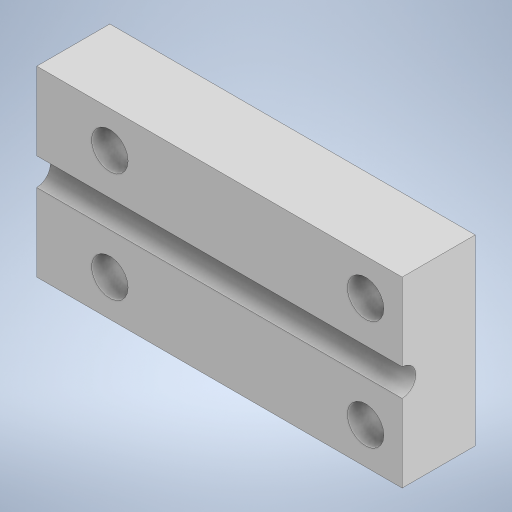
# Autodesk Inventor part: fiber_top
Saved by Autodesk Inventor 2024 (Build 280153000, 153)
## iProperties
Created: 2023-11-01
Part Number: fiber_top
Material: Generic
Document SubType Name: Modeling
Designer: toybox
Density: 1 g/cm^3
Appearance: Default
Author: toybox
Autodesk Inventor part; units mm, degrees
ref_plane "YZ Plane" through (0, 0, 0) normal (1, 0, 0) x (0, 1, 0)
ref_plane "XZ Plane" through (0, 0, 0) normal (0, 1, 0) x (-1, 0, 0)
ref_plane "XY Plane" through (0, 0, 0) normal (0, 0, 1) x (1, 0, 0)
sketch "Sketch3" plane through (0, 0, 0) normal (0, 0, 1) x (1, 0, 0)
  line L0 (-10, 5) -> (10, 5)
  line L1 (10, 5) -> (10, -5)
  line L2 (10, -5) -> (-10, -5)
  line L3 (-10, -5) -> (-10, 5)
  line L4 (-10, 5) -> (10, -5) construction
  line L5 (10, 5) -> (-10, -5) construction
  point P0 (0, 0)
  dimension "d5" = 20
  dimension "d6" = 10
  constraints: 12 end point, 2 midpoint, 2 parallel, 1 horizontal, 1 perpendicular
  measures "d5" distance of L1.end L2.end
  measures "d6" distance of L0.end L1.end
extrude "Extrusion2" add sketch "Sketch3" along normal blind 4
sketch "Sketch4" plane through (10, -5, 0) normal (1, 0, 0) x (0, 0, -1)
  circle A0 centre (-4, 5) radius 0.75
  point P0 (0, 5)
  dimension "d10" = 1.5
  constraints: 1 centre point
  measures "d10" diameter of A0
extrude "Extrusion3" cut sketch "Sketch4" against normal through all
sketch "Sketch5" plane through (0, 0, 4) normal (0, 0, 1) x (1, 0, 0)
  circle A0 centre (8, 3) radius 1
  circle A1 centre (8, -3) radius 1
  circle A2 centre (-6, 3) radius 1
  circle A3 centre (-6, -3) radius 1
  point P0 (0, 0)
  dimension "d17" = 2
  dimension "d16" = 2
  dimension "d15" = 2
  dimension "d14" = 2
  constraints: 4 centre point
  measures "d17" diameter of A0
  measures "d16" diameter of A1
  measures "d15" diameter of A2
  measures "d14" diameter of A3
extrude "Extrusion4" cut sketch "Sketch5" against normal through all
sketch "Sketch6" plane through (0, 0, 0) normal (0, 0, -1) x (-1, 0, 0)
  line L0 (-8.1739, 1.5824) -> (1.6987, 1.5824) construction
  line L1 (1.6987, 1.5824) -> (1.6987, -1.5298) construction
  line L2 (1.6987, -1.5298) -> (-8.1739, -1.5298) construction
  line L3 (-8.1739, -1.5298) -> (-8.1739, 1.5824) construction
  line L4 (-7.2861, -1.2743) -> (-7.2861, 1.3892)
  spline S0 degree 2 poles (-7.2861, 1.3892) (-7.2861, 1.5824) (-7.09, 1.5824) knots 0 0 0 1 1 1
  line L5 (-7.09, 1.5824) -> (-5.9053, 1.5824)
  spline S1 degree 2 poles (-5.9053, 1.5824) (-5.7093, 1.5824) (-5.7093, 1.3892) knots 0 0 0 1 1 1
  spline S2 degree 2 poles (-5.7093, 1.3892) (-5.7093, 1.1931) (-5.9053, 1.1931) knots 0 0 0 1 1 1
  line L6 (-5.9053, 1.1931) -> (-6.894, 1.1931)
  line L7 (-6.894, 1.1931) -> (-6.894, 0.3977)
  line L8 (-6.894, 0.3977) -> (-5.9053, 0.3977)
  spline S3 degree 2 poles (-5.9053, 0.3977) (-5.7093, 0.3977) (-5.7093, 0.2045) knots 0 0 0 1 1 1
  spline S4 degree 2 poles (-5.7093, 0.2045) (-5.7093, 0.0084) (-5.9053, 0.0084) knots 0 0 0 1 1 1
  line L9 (-5.9053, 0.0084) -> (-6.894, 0.0084)
  line L10 (-6.894, 0.0084) -> (-6.894, -1.2743)
  spline S5 degree 2 poles (-6.894, -1.2743) (-6.894, -1.4704) (-7.09, -1.4704) knots 0 0 0 1 1 1
  spline S6 degree 2 poles (-7.09, -1.4704) (-7.2861, -1.4704) (-7.2861, -1.2743) knots 0 0 0 1 1 1
  spline S7 degree 2 poles (-3.3734, 0.5014) (-3.3734, 0.6918) (-3.1774, 0.6918) knots 0 0 0 1 1 1
  spline S8 degree 2 poles (-3.1774, 0.6918) (-2.9813, 0.6918) (-2.9813, 0.5014) knots 0 0 0 1 1 1
  line L11 (-2.9813, 0.5014) -> (-2.9813, -1.2743)
  spline S9 degree 2 poles (-2.9813, -1.2743) (-2.9813, -1.4704) (-3.1774, -1.4704) knots 0 0 0 1 1 1
  spline S10 degree 2 poles (-3.1774, -1.4704) (-3.3734, -1.4704) (-3.3734, -1.2743) knots 0 0 0 1 1 1
  line L12 (-3.3734, -1.2743) -> (-3.3734, 0.5014)
  line L13 (-3.3734, 1.2379) -> (-3.3734, 1.3864)
  spline S11 degree 2 poles (-3.3734, 1.3864) (-3.3734, 1.5796) (-3.1774, 1.5796) knots 0 0 0 1 1 1
  spline S12 degree 2 poles (-3.1774, 1.5796) (-2.9813, 1.5796) (-2.9813, 1.3864) knots 0 0 0 1 1 1
  line L14 (-2.9813, 1.3864) -> (-2.9813, 1.2379)
  spline S13 degree 2 poles (-2.9813, 1.2379) (-2.9813, 1.0447) (-3.1774, 1.0447) knots 0 0 0 1 1 1
  spline S14 degree 2 poles (-3.1774, 1.0447) (-3.3734, 1.0447) (-3.3734, 1.2379) knots 0 0 0 1 1 1
  line L15 (0.9313, 0.0588) -> (0.9313, -0.8318)
  spline S15 degree 2 poles (0.9313, -0.8318) (0.9313, -1.1007) (0.5616, -1.4704) (0.2927, -1.4704) knots 0 0 0 1 2 2 2
  line L16 (0.2927, -1.4704) -> (-0.4467, -1.4704)
  spline S16 degree 2 poles (-0.4467, -1.4704) (-0.6427, -1.4704) (-0.6427, -1.2743) knots 0 0 0 1 1 1
  line L17 (-0.6427, -1.2743) -> (-0.6427, 1.3864)
  spline S17 degree 2 poles (-0.6427, 1.3864) (-0.6427, 1.5796) (-0.4467, 1.5796) knots 0 0 0 1 1 1
  spline S18 degree 2 poles (-0.4467, 1.5796) (-0.2506, 1.5796) (-0.2506, 1.3864) knots 0 0 0 1 1 1
  line L18 (-0.2506, 1.3864) -> (-0.2506, 0.6946)
  line L19 (-0.2506, 0.6946) -> (0.2927, 0.6946)
  spline S19 degree 2 poles (0.2927, 0.6946) (0.6652, 0.6946) (0.8473, 0.3781) knots 0 0 0 1 1 1
  spline S20 degree 2 poles (0.8473, 0.3781) (0.9313, 0.2297) (0.9313, 0.0588) knots 0 0 0 1 1 1
  line L20 (0.2927, 0.3053) -> (-0.2506, 0.3053)
  line L21 (-0.2506, 0.3053) -> (-0.2506, -1.0811)
  line L22 (-0.2506, -1.0811) -> (0.2927, -1.0811)
  spline S21 degree 2 poles (0.2927, -1.0811) (0.3935, -1.0811) (0.5392, -0.9354) (0.5392, -0.829) knots 0 0 0 1 2 2 2
  line L23 (0.5392, -0.829) -> (0.5392, 0.056)
  spline S22 degree 2 poles (0.5392, 0.056) (0.5392, 0.1625) (0.3963, 0.3053) (0.2927, 0.3053) knots 0 0 0 1 2 2 2
  line L24 (3.071, -0.5825) -> (3.071, -0.829)
  spline S23 degree 2 poles (3.071, -0.829) (3.071, -0.9326) (3.2195, -1.0811) (3.3203, -1.0811) knots 0 0 0 1 2 2 2
  line L25 (3.3203, -1.0811) -> (4.0597, -1.0811)
  spline S24 degree 2 poles (4.0597, -1.0811) (4.2558, -1.0811) (4.2558, -1.2743) knots 0 0 0 1 1 1
  spline S25 degree 2 poles (4.2558, -1.2743) (4.2558, -1.4704) (4.0597, -1.4704) knots 0 0 0 1 1 1
  line L26 (4.0597, -1.4704) -> (3.3203, -1.4704)
  spline S26 degree 2 poles (3.3203, -1.4704) (3.0486, -1.4704) (2.6789, -1.1007) (2.6789, -0.8318) knots 0 0 0 1 2 2 2
  line L27 (2.6789, -0.8318) -> (2.6789, -0.0924)
  spline S27 degree 2 poles (2.6789, -0.0924) (2.6789, 0.2325) (3.1383, 0.6918) (3.4659, 0.6918) knots 0 0 0 1 2 2 2
  spline S28 degree 2 poles (3.4659, 0.6918) (3.7992, 0.6918) (4.2558, 0.2381) (4.2558, -0.0924) knots 0 0 0 1 2 2 2
  line L28 (4.2558, -0.0924) -> (4.2558, -0.5825)
  line L29 (4.2558, -0.5825) -> (3.071, -0.5825)
  spline S29 degree 2 poles (3.4659, 0.3053) (3.3035, 0.3053) (3.071, 0.0728) (3.071, -0.0896) knots 0 0 0 1 2 2 2
  line L30 (3.071, -0.0896) -> (3.071, -0.1932)
  line L31 (3.071, -0.1932) -> (3.8636, -0.1932)
  line L32 (3.8636, -0.1932) -> (3.8636, -0.0896)
  spline S30 degree 2 poles (3.8636, -0.0896) (3.8636, 0.0728) (3.6312, 0.3053) (3.4659, 0.3053) knots 0 0 0 1 2 2 2
  spline S31 degree 2 poles (6.149, 0.5014) (6.149, 0.6946) (6.3451, 0.6946) knots 0 0 0 1 1 1
  line L33 (6.3451, 0.6946) -> (7.2329, 0.6946)
  spline S32 degree 2 poles (7.2329, 0.6946) (7.429, 0.6946) (7.429, 0.5014) knots 0 0 0 1 1 1
  line L34 (7.429, 0.5014) -> (7.429, 0.2045)
  spline S33 degree 2 poles (7.429, 0.2045) (7.429, 0.0084) (7.2329, 0.0084) knots 0 0 0 1 1 1
  spline S34 degree 2 poles (7.2329, 0.0084) (7.0369, 0.0084) (7.0369, 0.2045) knots 0 0 0 1 1 1
  line L35 (7.0369, 0.2045) -> (7.0369, 0.3053)
  line L36 (7.0369, 0.3053) -> (6.5412, 0.3053)
  line L37 (6.5412, 0.3053) -> (6.5412, -1.2743)
  spline S35 degree 2 poles (6.5412, -1.2743) (6.5412, -1.4704) (6.3451, -1.4704) knots 0 0 0 1 1 1
  spline S36 degree 2 poles (6.3451, -1.4704) (6.149, -1.4704) (6.149, -1.2743) knots 0 0 0 1 1 1
  line L38 (6.149, -1.2743) -> (6.149, 0.5014)
  point P0 (0, 0)
  constraints: 2 other
extrude "Extrusion5" cut sketch "Sketch6" against normal blind 0.5
body "Solid2"
